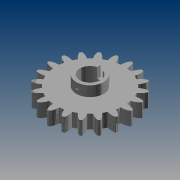
# Autodesk Inventor part: Part1
Saved by Autodesk Inventor 2014 (Build 180170000, 170)
## iProperties
Created: 2021-03-18
Part Number: Part1
Material: Stainless Steel
Document SubType Name: Modeling
Designer: Think Station
Density: 8.08 g/cm^3
Appearance: Semi-Polished
Author: Think Station
Autodesk Inventor part; units mm, degrees
ref_plane "YZ Plane" through (0, 0, 0) normal (1, 0, 0) x (0, 1, 0)
ref_plane "XY Plane" through (0, 0, 0) normal (0, 0, 1) x (1, 0, 0)
sketch "Sketch1" plane through (0, 0, 0) normal (0, 0, 1) x (1, 0, 0)
  circle A0 centre (0, 0) radius 50
  dimension "d0" = 100
  constraints: 1 centre point, 1 coincident
  measures "d0" diameter of A0
extrude "Extrusion1" add sketch "Sketch1" along normal blind 20
sketch "Sketch2" plane through (0, 0, 20) normal (0, 0, 1) x (1, 0, 0)
  circle A0 centre (0, 0) radius 50 projected
  line L0 (-1.5, 61.7971) -> (1.5, 61.7971)
  line L1 (-4.5, 49.7971) -> (4.5, 49.7971)
  arc A1 (-1.5, 61.7971) -> (-4.5, 49.7971) centre (15.4518, 51.1841) ccw
  arc A2 (4.5, 49.7971) -> (1.5, 61.7971) centre (-15.4518, 51.1841) ccw
  dimension "d5" = 3
  dimension "d6" = 9
  dimension "d7" = 20
  dimension "d8" = 20
  dimension "d9" = 12
  dimension "d10" = 3
  constraints: 6 point on circle, 4 end point, 2 centre point, 1 horizontal, 1 parallel
  measures "d5" distance of L0.start L0.end
  measures "d6" distance of L1.start L1.end
  measures "d7" radius of A1
  measures "d8" radius of A2
  measures "d9" distance between parallel lines of L1 L0
  measures "d10" horizontal distance of L1.start L0.start
extrude "Extrusion2" add sketch "Sketch2" against normal blind 20 contours A0 A1 L0 A2
fillet "Fillet1" radius 1 2 edges at (-1.5, 61.7971, 10) (1.5, 61.7971, 10)
fillet "Fillet2" radius 1 2 edges at (4.5, 49.7971, 10) (-4.5, 49.7971, 10)
pattern_circular "Circular Pattern1" count 20 over 360 about axis through (0, 0, 0) along (0, 0, 1) of "Extrusion2", "Fillet1", "Fillet2"
sketch "Sketch3" plane through (0, 0, 20) normal (0, 0, 1) x (1, 0, 0)
  arc A0 (10.1914, 48.9503) -> (5.4338, 49.7039) centre (0, 0) ccw projected
  circle A1 centre (0, 0) radius 20
  circle A2 centre (0, 0) radius 15
  dimension "d18" = 40
  dimension "d19" = 30
  constraints: 2 centre point, 2 coincident
  measures "d18" diameter of A1
  measures "d19" diameter of A2
extrude "Extrusion3" add sketch "Sketch3" along normal blind 15 and the other way blind 25
sketch "Sketch4" plane through (0, 0, 20) normal (0, 0, 1) x (1, 0, 0)
  circle A0 centre (0, 0) radius 15 projected
  circle A1 centre (0, 0) radius 15 projected
extrude "Extrusion4" cut sketch "Sketch4" against normal blind 30
sketch "Sketch5" plane through (0, 0, 35) normal (0, 0, 1) x (1, 0, 0)
  circle A0 centre (0, 0) radius 15 projected
  circle A1 centre (0, 0) radius 20 projected
  line L0 (4, 14.4568) -> (4, 19.5959)
  line L1 (-4, 19.5959) -> (-4, 14.4568)
  arc A2 (4, 19.5959) -> (-4, 19.5959) centre (0, 0) ccw
  arc A3 (4, 14.4568) -> (-4, 14.4568) centre (0, 0) ccw
  constraints: 8 point on circle, 4 end point, 2 centre point, 2 concentric, 1 parallel
extrude "Extrusion5" cut sketch "Sketch5" against normal blind 15 contours A0 L1 A1 L0 picked at (3.1159, 16.3307)
ref_plane "Work Plane1" through (0, -20, 0) normal (0, 1, 0) x (-1, 0, 0)
sketch "Sketch6" plane through (0, -20, 0) normal (0, 1, 0) x (-1, 0, 0)
  circle A0 centre (0, 27.5) radius 2.5
  line L0 (20, 35) -> (-20, 35) projected
  line L1 (20, 20) -> (20, 35) projected
  point P0 (0, 0)
  point P1 (4, 35)
  point P2 (-4, 35)
  dimension "d30" = 5
  dimension "d31" = 7.5
  dimension "d32" = 20
  constraints: 1 centre point
  measures "d30" diameter of A0
  measures "d31" distance from line of A0.centre L0
  measures "d32" distance from line of L1 A0.centre
extrude "Extrusion6" cut sketch "Sketch6" along normal blind 15
thread "Thread1" size "M5x0.8" class "6H" standard "ANSI Metric M Profile" full length
body "Solid1"
